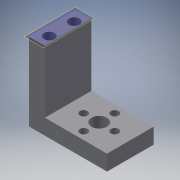
# Autodesk Inventor part: base_bracket
Saved by Autodesk Inventor 2016 (Build 200138000, 138)
## iProperties
Created: 2016-01-27
Part Number: base_bracket
Material: Generic
Document SubType Name: Modeling
Designer: seve
Density: 1 g/cm^3
Appearance: Default
Author: seve
Autodesk Inventor part; units mm, degrees
ref_plane "YZ Plane" through (0, 0, 0) normal (1, 0, 0) x (0, 1, 0)
ref_plane "XZ Plane" through (0, 0, 0) normal (0, 1, 0) x (-1, 0, 0)
ref_plane "XY Plane" through (0, 0, 0) normal (0, 0, 1) x (1, 0, 0)
ref_plane "Work Plane1" through (-67.6204, 38.5563, -2.9554) normal (0, -1, 0) x (1, 0, 0)
sketch "Sketch1" plane through (-67.6204, 38.5563, -2.9554) normal (0, -1, 0) x (1, 0, 0)
  arc A0 (50.3009, 14.0884) -> (50.3009, 11.4884) centre (48.5884, 12.7884) ccw projected
  arc A1 (50.3009, 3.8884) -> (50.3009, 1.2884) centre (48.5884, 2.5884) ccw projected
  circle A2 centre (48.5884, 12.7884) radius 2.15
  circle A3 centre (48.5884, 2.5884) radius 2.15
  line L0 (44.6884, 13.4384) -> (44.6884, 1.9384) projected
  line L1 (51.1884, 3.8884) -> (51.1884, 11.4884) projected
  line L2 (49.3768, 17.1884) -> (44.0113, 17.1884) projected
  line L3 (44.0113, -1.8116) -> (49.3768, -1.8116) projected
  line L4 (51.1884, 17.1884) -> (44.6884, 17.1884)
  line L5 (44.6884, 17.1884) -> (44.6884, -1.8116)
  line L6 (44.6884, -1.8116) -> (51.1884, -1.8116)
  line L7 (51.1884, -1.8116) -> (51.1884, 17.1884)
  point P0 (67.6204, 2.9554)
  constraints: 8 end point, 2 centre point, 2 coincident, 2 concentric, 2 parallel, 1 horizontal, 1 perpendicular, 1 point on line
extrude "Extrusion1" add sketch "Sketch1" along normal blind 31.75
sketch "Sketch2" plane through (-16.432, 38.5563, 14.233) normal (1, 0, 0) x (0, 0, -1)
  line L0 (19, 0) -> (19, -31.75) projected
  line L1 (0, -31.75) -> (19, -31.75)
  line L2 (19, -31.75) -> (19, -25.4)
  line L3 (19, -25.4) -> (0, -25.4)
  line L4 (0, -25.4) -> (0, -31.75)
  point P0 (14.233, -38.5563)
  dimension "d2" = 6.35
  constraints: 8 end point, 2 parallel, 1 horizontal, 1 perpendicular, 1 point on line
  measures "d2" distance between parallel lines of L1 L3
extrude "Extrusion2" add sketch "Sketch2" along normal blind 25.4
sketch "Sketch3" plane through (-16.432, 13.1563, 14.233) normal (0, 1, 0) x (1, 0, 0)
  line L0 (0, 19) -> (25.4, 19) projected
  line L1 (25.4, 19) -> (25.4, 0) projected
  point P0 (16.432, 14.233)
  point P1 (12.7, 9.5)
hole "Hole1" at (-3.732, 13.1563, 4.733) direction (0, -1, 0) diameter 6.35 end through all
sketch "Sketch4" plane through (-16.432, 13.1563, 14.233) normal (0, 1, 0) x (1, 0, 0)
  circle A0 centre (12.7, 9.5) radius 3.175 projected
  point P0 (16.432, 14.233)
  point P1 (6.35, 9.5)
  point P2 (12.7, 3.15)
  point P3 (19.05, 9.5)
  point P4 (12.7, 15.85)
  dimension "d12" = 6.35
  dimension "d15" = 360
  constraints: 5 other
  measures "d12" distance of A0.centre point (6.35, 9.5)
hole "Hole2" at (-10.082, 13.1563, 4.733) at (-3.732, 13.1563, 11.083) at (2.618, 13.1563, 4.733) at (-3.732, 13.1563, -1.617) direction (0, -1, 0) diameter 3.175 end through all
body "Solid1"
